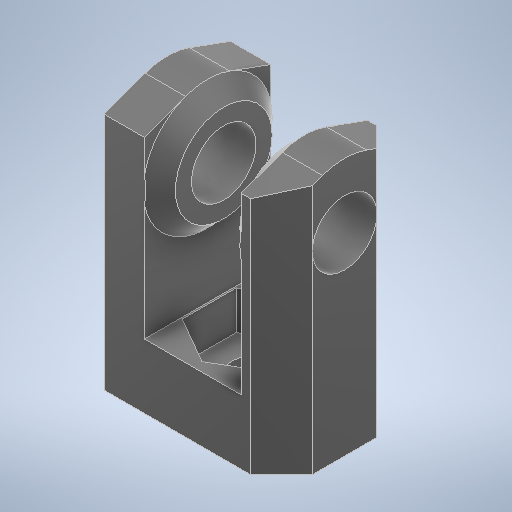
# Autodesk Inventor part: Tensioner
Saved by Autodesk Inventor 2026.2 (Build 302298000, 298)
## iProperties
Created: 2026-03-30
Part Number: Tensioner
Material: ABS Plastic
Document SubType Name: Modeling
Designer: gaoet
Density: 1.06 g/cm^3
Appearance: Smooth - Black
Author: gaoet
Autodesk Inventor part; units mm, degrees
ref_plane "YZ Plane" through (0, 0, 0) normal (1, 0, 0) x (0, 1, 0)
ref_plane "XZ Plane" through (0, 0, 0) normal (0, 1, 0) x (-1, 0, 0)
ref_plane "XY Plane" through (0, 0, 0) normal (0, 0, 1) x (1, 0, 0)
sketch "Sketch1" plane through (0, 0, 0) normal (0, 0, 1) x (1, 0, 0)
  line L0 (-5.5, -8) -> (5.5, -8)
  line L1 (5.5, -8) -> (5.5, 8)
  line L2 (5.5, 8) -> (-5.5, 8)
  line L3 (-5.5, 8) -> (-5.5, -8)
  line L4 (-5.5, -8) -> (5.5, 8) construction
  line L5 (5.5, -8) -> (-5.5, 8) construction
  line L6 (-3, 8) -> (3, 8)
  line L7 (3, 8) -> (3, -4)
  line L8 (3, -4) -> (-3, -4)
  line L9 (-3, -4) -> (-3, 8)
  point P0 (0, 0)
  dimension "d0" = 6
  dimension "d1" = 2.5
  dimension "d2" = 2.5
  dimension "d3" = 12
  dimension "d4" = 4
  constraints: 20 end point, 4 parallel, 2 horizontal, 2 midpoint, 2 perpendicular, 1 point on line
  measures "d0" distance of L7.end L8.end
  measures "d1" distance between parallel lines of L3 L9
  measures "d2" distance between parallel lines of L7 L1
  measures "d3" distance of L6.end L7.end
  measures "d4" distance between parallel lines of L0 L8
extrude "Extrusion1" add sketch "Sketch1" along normal blind 8 contours L3 L2 L9 L8 L7 L1 L0
sketch "Sketch2" plane through (-5.5, -8, 0) normal (-1, 0, 0) x (0, 0, 1)
  circle A0 centre (4, 12) radius 6.5
  line L0 (8, 16) -> (8, 0) projected
  line L1 (0, 16) -> (0, 0) projected
  line L2 (0, 4) -> (8, 4) projected
  line L3 (0, 16) -> (8, 16) projected
  point P0 (0, 8)
  dimension "d7" = 13
  dimension "d8" = 8
  dimension "d9" = 4
  dimension "d10" = 4
  constraints: 1 centre point
  measures "d7" diameter of A0
  measures "d8" distance between parallel lines of L0 L1
  measures "d9" distance from line of L1 A0.centre
  measures "d10" distance from line of L3 A0.centre
hole "Hole1" at (-5.5, 4, 4) direction (1, 0, 0) diameter 4 depth 50
sketch "Sketch3" plane through (-3, -4, 0) normal (0, 1, 0) x (1, 0, 0)
  line L0 (6, 0) -> (0, 0) projected
  line L1 (0, 0) -> (0, -8) projected
  line L2 (6, -8) -> (0, -8) projected
  line L3 (6, 0) -> (6, -8) projected
  line L4 (0.1, -2.3257) -> (3, -0.6514)
  line L5 (3, -0.6514) -> (5.9, -2.3257)
  line L6 (5.9, -2.3257) -> (5.9, -5.6743)
  line L7 (5.9, -5.6743) -> (3, -7.3486)
  line L8 (3, -7.3486) -> (0.1, -5.6743)
  line L9 (0.1, -5.6743) -> (0.1, -2.3257)
  point P0 (3, 0)
  point P1 (3, -4)
  point P2 (0, -5.4053)
  point P3 (4.4, -5.4053)
  point P4 (4.4, -1.5947)
  point P5 (0, -1.5947)
  dimension "d18" = 5.8
  dimension "d19" = 4
  dimension "d20" = 8
  dimension "d21" = 6
  dimension "d22" = 3
  constraints: 12 end point, 1 vertical, 13 other
  measures "d18" distance between parallel lines of L6 L9
  measures "d19" distance from line of L0 point (3, -4)
  measures "d20" distance between parallel lines of L2 L0
  measures "d21" distance of L0.start L0.end
  measures "d22" distance from line of L1 point (3, -4)
extrude "Extrusion2" cut sketch "Sketch3" against normal blind 2.4 contours L4 L5 L6 L7 L8 L9
sketch "Sketch4" plane through (-3, -4, 0) normal (1, 0, 0) x (0, 0, -1)
  circle A0 centre (-4, 8) radius 2 projected
  line L0 (0, 0) -> (0, 12) projected
  line L1 (0, 12) -> (-8, 12) projected
  line L2 (-8, 0) -> (-8, 12) projected
  line L3 (0, 0) -> (-8, 0) projected
  circle A1 centre (-4, 8) radius 4
  point P0 (0, 4)
  constraints: 1 centre point, 1 coincident, 1 tangent
extrude "Extrusion3" add sketch "Sketch4" along normal blind 1 contours A1
mirror "Mirror1" about plane through (0, 0, 0) normal (1, 0, 0) of "Extrusion3"
sketch "Sketch5" plane through (-5.5, -8, 0) normal (-1, 0, 0) x (0, 0, 1)
  arc A0 (0, 12) -> (8, 12) centre (4, 12) ccw projected
  circle A1 centre (4, 12) radius 2 projected
  line L0 (0, 16) -> (0, 0) projected
  line L1 (0, 0) -> (8, 0) projected
  line L2 (8, 16) -> (8, 0) projected
  line L3 (0, 16) -> (8, 16) projected
  circle A2 centre (4, 12) radius 4 projected
  circle A3 centre (4, 12) radius 2 projected
  point P0 (0, 8)
  point P1 (4, 16)
extrude "Extrusion4" cut sketch "Sketch5" against normal through all contours L0 L3 A2 | A2 L3 L2
sketch "Sketch7" plane through (-2, -4, 0) normal (1, 0, 0) x (0, 0, -1)
  circle A0 centre (-4, 8) radius 4 projected
  circle A1 centre (-4, 8) radius 2 projected
  line L0 (-5.3681, 4.2412) -> (-8, 5.1992)
  line L1 (-8, 5.1992) -> (-8, 8)
  point P0 (0, 4)
  dimension "d32" = 70
  constraints: 4 end point, 2 point on circle, 2 tangent, 1 vertical
  measures "d32" angle of L1 L0
extrude "Extrusion6" add sketch "Sketch7" against normal up to surface (1 mm away) contours A0 L0 L1
mirror "Mirror3" about plane through (0, 0, 0) normal (1, 0, 0) of "Extrusion6"
sketch "Sketch9" plane through (5.5, -8, 8) normal (1, 0, 0) x (0, 0, -1)
  arc A0 (8, 12) -> (0, 12) centre (4, 12) ccw projected
  line L0 (0, 0) -> (0, 12) projected
  line L1 (8, 0) -> (0, 0) projected
  line L2 (8, 0) -> (8, 12) projected
  circle A1 centre (4, 12) radius 2 projected
  line L3 (2.6319, 15.7588) -> (0, 14.8008)
  line L4 (0, 14.8008) -> (0, 12)
  arc A2 (8, 12) -> (0, 12) centre (4, 12) ccw projected
  line L5 (8, 12) -> (8, 14.8008)
  line L6 (8, 14.8008) -> (5.3681, 15.7588)
  point P0 (8, 8)
  point P1 (5.3681, 15.7588)
  dimension "d42" = 70
  constraints: 8 end point, 3 point on circle, 3 tangent, 2 vertical, 1 equal length
  measures "d42" angle of L4 L3
extrude "Extrusion7" add sketch "Sketch9" against normal up to surface (3.5 mm away) contours A0 L6 L5 | A0 L4 L3
mirror "Mirror4" about plane through (0, 0, 0) normal (1, 0, 0) of "Extrusion7"
sketch "Sketch10" plane through (-2, -4, 0) normal (1, 0, 0) x (0, 0, -1)
  arc A0 (-5.3681, 4.2412) -> (0, 8) centre (-4, 8) ccw projected
  line L0 (-5.3681, 11.7588) -> (-8, 10.8008) projected
  line L1 (-8, 10.8008) -> (-8, 5.1992) projected
  line L2 (-8, 5.1992) -> (-5.3681, 4.2412) projected
  circle A1 centre (-4, 8) radius 2 projected
  circle A2 centre (-4, 8) radius 3
  line L3 (0, 8) -> (0, 10.8008) projected
  line L4 (0, 10.8008) -> (-2.6319, 11.7588) projected
  arc A3 (-2.6319, 11.7588) -> (-5.3681, 11.7588) centre (-4, 8) ccw projected
  point P0 (0, 4)
  dimension "d45" = 1
  constraints: 1 centre point
  measures "d45" radial gap between concentric circles of A2 A1
extrude "Extrusion8" cut sketch "Sketch10" against normal up to surface (1 mm away) contours L2 L1 L0 A3 L4 L3 A0
mirror "Mirror5" about plane through (0, 0, 0) normal (1, 0, 0) of "Extrusion8"
chamfer "Chamfer2" distance 1 angle 45 2 edges at (3, 4, 7) (-3, 4, 7)
sketch "Sketch11" plane through (-5.5, -8, 0) normal (0, -1, 0) x (1, 0, 0)
  line L0 (0, 0) -> (11, 0) projected
  line L1 (11, 0) -> (11, 8) projected
  line L2 (0, 8) -> (11, 8) projected
  line L3 (0, 0) -> (0, 8) projected
  line L4 (11, 8) -> (0, 8)
  line L5 (0, 8) -> (0, 0)
  line L6 (0, 0) -> (11, 0)
  line L7 (11, 0) -> (11, 8)
  line L8 (11, 8) -> (0, 0) construction
  line L9 (0, 8) -> (11, 0) construction
  point P0 (5.5, 0)
  point P1 (5.5, 4)
  constraints: 12 end point, 2 collinear, 2 midpoint, 2 parallel, 1 horizontal, 1 perpendicular
hole "Hole3" at (0, -8, 4) direction (0, 1, 0) diameter 3 depth 50
chamfer "Chamfer3" distance 2 angle 45 2 edges at (5.5, -0.5996, 8) (5.5, -0.5996, 0)
sketch "Sketch12" plane through (-5.5, -8, 0) normal (0, -1, 0) x (1, 0, 0)
  line L0 (11, 2) -> (9, 0) projected
  line L1 (11, 2) -> (11, 6) projected
  line L2 (9, 8) -> (11, 6) projected
  line L3 (0, 8) -> (9, 8) projected
  line L4 (0, 0) -> (0, 8) projected
  line L5 (0, 0) -> (9, 0) projected
  circle A0 centre (5.5, 4) radius 1.5 projected
  line L6 (8.9669, 0.08) -> (10.92, 2.0331)
  line L7 (10.92, 2.0331) -> (10.92, 5.9669)
  line L8 (10.92, 5.9669) -> (8.9669, 7.92)
  line L9 (8.9669, 7.92) -> (0.08, 7.92)
  line L10 (0.08, 7.92) -> (0.08, 0.08)
  line L11 (0.08, 0.08) -> (8.9669, 0.08)
  line L12 (0.08, 0.08) -> (0, 0.08)
  line L13 (0.08, 7.92) -> (0, 7.92)
  line L14 (8.9669, 0.08) -> (9.08, 0.08)
  line L15 (8.9669, 7.92) -> (9.08, 7.92)
  point P0 (5.5, 0)
  dimension "d64" = 0.08
  constraints: 20 end point, 4 point on line, 2 horizontal, 1 parallel, 1 perpendicular, 5 other
  measures "d64" distance between parallel lines of L11 L5
extrude "Extrusion9" cut sketch "Sketch12" against normal through all contours L0 L5 L4 L12 L11 L14 | L15 L9 L13 L4 L3 L2
equation "\"d2\" = d1"
equation "\"d9\" = 0.5 * d8"
equation "\"d19\" = 0.5 * d20"
equation "\"d22\" = 0.5 * d21"
body "Solid1"
